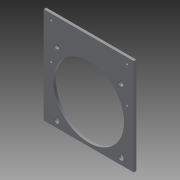
# Autodesk Inventor part: base_usb3
Saved by Autodesk Inventor 2014 (Build 180170000, 170)
## iProperties
Created: 2015-04-20
Part Number: base_usb3
Material: Generic
Document SubType Name: Modeling
Designer: Sousaadm
Density: 1 g/cm^3
Appearance: Default
Author: Sousaadm
Autodesk Inventor part; units mm, degrees
ref_plane "YZ Plane" through (0, 0, 0) normal (1, 0, 0) x (0, 1, 0)
ref_plane "XZ Plane" through (0, 0, 0) normal (0, 1, 0) x (-1, 0, 0)
ref_plane "XY Plane" through (0, 0, 0) normal (0, 0, 1) x (1, 0, 0)
sketch "Sketch1" plane through (0, 0, 0) normal (0, 1, 0) x (-1, 0, 0)
  line L0 (0, 0) -> (-70, 0)
  line L1 (-70, 0) -> (-70, 75)
  line L2 (-70, 75) -> (0, 75)
  line L3 (0, 75) -> (0, 0)
  dimension "d0" = 75
  dimension "d1" = 70
  constraints: 8 end point, 2 parallel, 1 horizontal, 1 perpendicular
  measures "d0" distance of L2.end L0.start
  measures "d1" distance of L1.end L2.end
extrude "Extrusion1" add sketch "Sketch1" along normal blind 2
sketch "Sketch2" plane through (0, 0, 0) normal (0, -1, 0) x (1, 0, 0)
  line L0 (70, 0) -> (70, 75) projected
  line L1 (70, 75) -> (0, 75) projected
  circle A0 centre (60, 55) radius 2
  circle A1 centre (10, 55) radius 2
  circle A2 centre (60, 5) radius 2
  circle A3 centre (10, 5) radius 2
  line L2 (0, 0) -> (70, 0) projected
  line L3 (35, 75) -> (35, 0) construction
  line L4 (5, 0) -> (65, 0) construction
  line L5 (65, 0) -> (65, 60) construction
  line L6 (65, 60) -> (5, 60) construction
  line L7 (5, 60) -> (5, 0) construction
  line L8 (5, 0) -> (65, 60) construction
  line L9 (65, 0) -> (5, 60) construction
  circle A4 centre (35, 30) radius 27.5
  dimension "d7" = 4
  dimension "d44" = 50
  dimension "d47" = 50
  dimension "d56" = 55
  dimension "d71" = 60
  dimension "d72" = 60
  dimension "d73" = 30
  dimension "d74" = 5
  dimension "d75" = 55
  constraints: 14 end point, 5 centre point, 4 midpoint, 2 horizontal, 2 parallel, 1 coincident, 1 perpendicular, 1 point on line, 1 vertical, 6 other
  measures "d7" diameter of A0
  measures "d44" distance of A0.centre A1.centre
  measures "d47" distance of A0.centre A2.centre
  measures "d56" distance from line of L2 A0.centre
  measures "d71" distance of L4.end L5.end
  measures "d72" distance of L5.end L6.end
  measures "d73" distance from line of L2 point (35, 30)
  measures "d74" distance from line of L5 A0.centre
  measures "d75" diameter of A4
extrude "Extrusion2" cut sketch "Sketch2" against normal through all
sketch "Sketch5" plane through (0, 0, 0) normal (0, -1, 0) x (1, 0, 0)
  line L0 (0, 0) -> (70, 0) projected
  line L1 (70, 0) -> (70, 75) projected
  line L2 (70, 75) -> (0, 75) projected
  circle A0 centre (64.5, 70.5) radius 1
  circle A1 centre (5.5, 70.5) radius 1
  circle A2 centre (64.5, 42.5) radius 1
  circle A3 centre (5.5, 42.5) radius 1
  line L3 (35, 75) -> (35, 0) construction
  dimension "d57" = 2
  dimension "d58" = 4.5
  dimension "d61" = 59
  dimension "d64" = 28
  dimension "d68" = 59
  constraints: 4 centre point, 2 end point, 2 midpoint, 1 horizontal, 1 vertical, 6 other
  measures "d57" diameter of A0
  measures "d58" distance from line of L2 A0.centre
  measures "d61" distance of A0.centre A1.centre
  measures "d64" distance of A0.centre A2.centre
  measures "d68" diameter of A0.centre L3
extrude "Extrusion5" cut sketch "Sketch5" against normal through all
body "Solid1"
